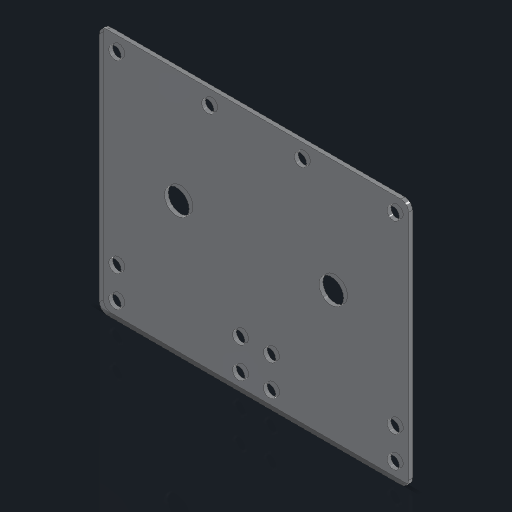
# Autodesk Inventor part: Polycarbonate Kicker plate
Saved by Autodesk Inventor 2023.2 (Build 272271030, 271C)
## iProperties
Created: 2023-12-10
Part Number: Polycarbonate Kicker plate
Material: Polycarbonate, Clear
Document SubType Name: Modeling
Designer: Michael
Density: 1.2 g/cm^3
Appearance: Polycarbonate - Clear
Mass: 23.7919 g
Surface Area: 261.009 cm^2
Volume: 19.8266 cm^3
Author: Michael
Autodesk Inventor part; units mm, degrees
ref_plane "YZ Plane" through (0, 0, 0) normal (1, 0, 0) x (0, 1, 0)
ref_plane "XZ Plane" through (0, 0, 0) normal (0, 1, 0) x (-1, 0, 0)
ref_plane "XY Plane" through (0, 0, 0) normal (0, 0, 1) x (1, 0, 0)
sketch "Sketch1" plane through (0, 0, 0) normal (0, 0, 1) x (1, 0, 0)
  line L0 (0, 0) -> (-127, 0)
  line L1 (-127, 0) -> (-127, 101.6)
  line L2 (-127, 101.6) -> (0, 101.6)
  line L3 (0, 101.6) -> (0, 0)
  dimension "d0" = 127
  dimension "d1" = 101.6
  constraints: 8 end point, 2 parallel, 1 horizontal, 1 perpendicular
  measures "d0" distance of L1.end L2.end
  measures "d1" distance of L0.end L1.end
extrude "Extrusion1" add sketch "Sketch1" along normal blind 1.5875
sketch "Sketch3" plane through (0, 0, 1.5875) normal (0, 0, 1) x (1, 0, 0)
  line L0 (0, 101.6) -> (-127, 101.6) projected
  line L1 (-6.35, 101.6) -> (-6.35, 95.25)
  line L2 (-6.35, 95.25) -> (0, 95.25)
  line L3 (0, 0) -> (0, 101.6) projected
  line L4 (-6.35, 95.25) -> (-44.45, 95.25)
  line L5 (-44.45, 95.25) -> (-82.55, 95.25)
  line L6 (-82.55, 95.25) -> (-120.65, 95.25)
  line L7 (-120.65, 95.25) -> (-127, 95.25)
  line L8 (-120.65, 95.25) -> (-120.65, 19.05)
  line L9 (-120.65, 19.05) -> (-120.65, 6.35)
  circle A0 centre (-120.65, 19.05) radius 2.54
  circle A1 centre (-120.65, 6.35) radius 2.54
  line L10 (-6.35, 95.25) -> (-6.35, 19.05)
  circle A2 centre (-6.35, 19.05) radius 2.54
  line L11 (-6.35, 19.05) -> (-6.35, 6.35)
  circle A3 centre (-6.35, 6.35) radius 2.54
  line L12 (-6.35, 6.35) -> (-57.15, 6.35)
  circle A4 centre (-57.15, 6.35) radius 2.54
  line L13 (-57.15, 6.35) -> (-69.85, 6.35)
  circle A5 centre (-69.85, 6.35) radius 2.54
  line L14 (-69.85, 6.35) -> (-120.65, 6.35)
  line L15 (-69.85, 6.35) -> (-69.85, 19.05)
  line L16 (-57.15, 6.35) -> (-57.15, 19.05)
  circle A6 centre (-69.85, 19.05) radius 2.54
  circle A7 centre (-57.15, 19.05) radius 2.54
  line L17 (-120.65, 95.25) -> (-107.9525, 95.25)
  line L18 (-101.6, 95.25) -> (-95.25, 95.25)
  line L19 (-95.25, 95.25) -> (-95.25, 54.61)
  circle A8 centre (-95.25, 54.61) radius 5.08
  line L20 (-25.4, 95.25) -> (-31.75, 95.25)
  line L21 (-44.45, 95.25) -> (-31.75, 95.25)
  line L22 (-31.75, 95.25) -> (-31.75, 54.61)
  circle A9 centre (-31.75, 54.61) radius 5.08
  line L23 (-120.65, 95.25) -> (-120.65, 97.79)
  line L24 (-6.35, 95.25) -> (-6.35, 97.79)
  line L25 (-82.55, 95.25) -> (-82.55, 97.79)
  line L26 (-44.45, 95.25) -> (-44.45, 97.79)
  line L27 (-120.65, 97.79) -> (-120.65, 96.52)
  line L28 (-82.55, 97.79) -> (-82.55, 96.52)
  line L29 (-44.45, 97.79) -> (-44.45, 96.52)
  line L30 (-6.35, 97.79) -> (-6.35, 96.52)
  line L31 (-120.65, 96.52) -> (-120.65, 94.9198)
  circle A10 centre (-120.65, 94.9198) radius 2.54
  line L32 (-82.55, 96.52) -> (-82.55, 94.9198)
  circle A11 centre (-82.55, 94.9198) radius 2.54
  line L33 (-44.45, 96.52) -> (-44.45, 94.9198)
  line L34 (-6.35, 96.52) -> (-6.35, 94.9198)
  circle A12 centre (-6.35, 94.9198) radius 2.54
  circle A13 centre (-44.45, 94.9198) radius 2.54
  dimension "d4" = 6.35
  dimension "d5" = 6.35
  dimension "d7" = 38.1
  dimension "d8" = 38.1
  dimension "d9" = 38.1
  dimension "d10" = 6.35
  dimension "d20" = 76.2
  dimension "d21" = 12.7
  dimension "d22" = 5.08
  dimension "d23" = 5.08
  dimension "d26" = 76.2
  dimension "d27" = 5.08
  dimension "d28" = 12.7
  dimension "d29" = 5.08
  dimension "d33" = 50.8
  dimension "d34" = 5.08
  dimension "d35" = 12.7
  dimension "d36" = 5.08
  dimension "d37" = 12.7
  dimension "d38" = 5.08
  dimension "d39" = 5.08
  dimension "d41" = 10.16
  dimension "d42" = 10.16
  dimension "d43" = 40.64
  dimension "d44" = 40.64
  dimension "d53" = 1.6002
  dimension "d54" = 5.08
  dimension "d55" = 1.6002
  dimension "d56" = 5.08
  dimension "d57" = 1.6002
  dimension "d58" = 1.6002
  dimension "d59" = 5.08
  dimension "d60" = 5.08
  constraints: 66 end point, 26 coincident, 14 centre point, 14 point on line, 8 vertical, 6 midpoint, 4 horizontal, 2 perpendicular, 1 collinear
  measures "d4" distance of L1.start L1.end
  measures "d5" distance of L1.end L2.end
  measures "d7" distance of L4.start L4.end
  measures "d8" distance of L4.end L5.end
  measures "d9" distance of L5.end L6.end
  measures "d10" distance of L6.end L7.end
  measures "d20" distance of L8.start L8.end
  measures "d21" distance of L8.end L9.end
  measures "d22" diameter of A0
  measures "d23" diameter of A1
  measures "d26" distance of L4.start L10.end
  measures "d27" diameter of A2
  measures "d28" distance of L11.start L11.end
  measures "d29" diameter of A3
  measures "d33" distance of L12.start L12.end
  measures "d34" diameter of A4
  measures "d35" distance of L13.start L13.end
  measures "d36" diameter of A5
  measures "d37" distance of L14.start L15.end
  measures "d38" diameter of A6
  measures "d39" diameter of A7
  measures "d41" diameter of A8
  measures "d42" diameter of A9
  measures "d43" distance of L18.end L19.end
  measures "d44" distance of L20.end L22.end
  measures "d53" distance of L31.start L31.end
  measures "d54" diameter of A10
  measures "d55" distance of L32.start L32.end
  measures "d56" diameter of A11
  measures "d57" distance of L33.start L33.end
  measures "d58" distance of L34.start L34.end
  measures "d59" diameter of A12
  measures "d60" diameter of A13
extrude "Extrusion2" cut sketch "Sketch3" against normal blind 25.4 contours A12 L10 L2 | L2 L1 A12 | L1 L4 A12 | L10 A12 L4 | A9 | A8 | A6 | A7 | A2 L11 L10 | L10 L11 A2 | A13 L5 L4 | L4 L26 A13 | A3 L12 L11 | L11 L12 A3 | L5 A13 L26 | A4 L13 L12 | L12 L16 A4 | A11 L6 L5 | L5 L25 A11 | L13 A4 L16 | L6 A11 L25 | A5 L14 L13 | L13 L15 A5 | L14 A5 L15 | L14 L9 A1 | A1 L9 L14 | A0 L8 L9 | L9 L8 A0 | A10 L8 L6 | L6 L23 A10 | L8 A10 L7 | L7 A10 L23
fillet "Fillet1" radius 3.175 4 edges at (-127, 101.6, 0.7937) (0, 101.6, 0.7937) (0, 0, 0.7937) (-127, 0, 0.7937)
body "Solid1"
